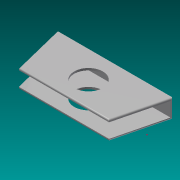
# Autodesk Inventor part: sambungan leaf spring
Saved by Autodesk Inventor 2014 SP2 (Build 180246200, 246)
## iProperties
Created: 2019-07-17
Part Number: sambungan leaf spring
Material: Steel, Mild
Document SubType Name: Modeling
Designer: USER PC
Density: 7.86 g/cm^3
Appearance: Steel
Mass: 1846.56 g
Surface Area: 1344.59 cm^2
Volume: 234.931 cm^3
Author: USER PC
Autodesk Inventor part; units mm, degrees
ref_plane "XZ Plane" through (0, 0, 0) normal (0, 1, 0) x (-1, 0, 0)
sketch "Sketch1" plane through (0, 0, 0) normal (0, 0, 1) x (1, 0, 0)
  circle A0 centre (0, 0) radius 35
  line L0 (0, 0) -> (0, 35)
  line L1 (0, 0) -> (0, -35)
  line L2 (110, -60) -> (141.25, 65)
  line L3 (-110, -60) -> (-141.25, 65)
  line L4 (0, -35) -> (0, -60)
  line L5 (0, -60) -> (110, -60)
  line L6 (0, -60) -> (-110, -60)
  line L7 (0, 35) -> (0, 65)
  line L8 (0, 65) -> (141.25, 65)
  line L9 (0, 65) -> (-141.25, 65)
  constraints: 20 end point, 3 collinear, 3 perpendicular, 2 point on circle, 1 centre point, 1 coincident, 1 vertical
extrude "Extrusion3" add sketch "Sketch1" along normal blind 45 contours A0 L7 L8 L2 L5 L4 | A0 L4 L6 L3 L9 L7
ref_plane "Work Plane2" through (142.5, 0, 0) normal (1, 0, 0) x (0, 1, 0)
fillet "Fillet2" radius 3 8 edges at (-141.25, 65, 22.5) (141.25, 65, 22.5) (125.625, 2.5, 45) (-125.625, 2.5, 45) (-125.625, 2.5, 0) (125.625, 2.5, 0) (0, -60, 0) (0, -60, 45)
sketch "Sketch5" plane through (142.5, 0, 0) normal (1, 0, 0) x (0, 1, 0)
  point P0 (0, 0)
ref_plane "Work Plane3" through (140, 0, 0) normal (1, 0, 0) x (0, 1, 0)
sketch "Sketch6" plane through (140, 0, 0) normal (1, 0, 0) x (0, 1, 0)
  line L0 (-56.5599, 40) -> (60, 40)
  line L1 (60, 40) -> (60, 5)
  line L2 (60, 5) -> (-60.1868, 5)
  line L3 (-56.5599, 40) -> (60, 5) construction
  line L4 (60, 40) -> (-60.1868, 5) construction
  line L5 (65, 0) -> (65, 45) projected
  line L6 (-56.5599, 40) -> (-64.3318, 40)
  line L7 (-64.3318, 40) -> (-64.3318, 5)
  line L8 (-64.3318, 5) -> (-60.1868, 5)
  line L9 (64.9104, 45) -> (-57, 45) projected
  line L10 (-57, 0) -> (64.9104, 0) projected
  point P0 (0, 0)
  point P1 (0.8272, 22.7681)
  dimension "d33" = 5
  dimension "d36" = 5
  dimension "d37" = 5
  constraints: 16 end point, 3 perpendicular, 2 parallel, 2 point on line, 1 horizontal
  measures "d33" distance between parallel lines of L5 L1
  measures "d36" distance between parallel lines of L9 L0
  measures "d37" distance between parallel lines of L2 L10
extrude "Extrusion5" cut sketch "Sketch6" against normal blind 1000
body "Solid2"
